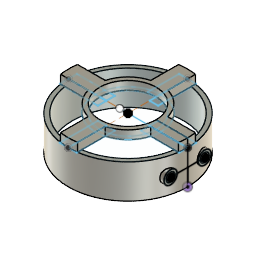
hexbug casing v6 (Autodesk Fusion 360 design; units mm, degrees)
Autodesk Fusion 360 part; units mm, degrees
sketch "Sketch1" plane through (0, 0, 0) normal (0, 0, 1) x (1, 0, 0)
  circle A0 centre (0, 0) radius 32.5
  circle A1 centre (0, 0) radius 35
  dimension "d1" = 65
  dimension "d2" = 70
  constraint coincident A0.centre A1.centre
  constraint concentric A0 A1
  measures "d1" diameter of A0
  measures "d2" diameter of A1
extrude "Extrude1" add sketch "Sketch1" along normal blind 20 makes body 1
sketch "Sketch2" plane through (0, 0, 0) normal (1, 0, 0) x (0, 1, 0)
  line L0 (0, 0) -> (0, 50)
  line L1 (0, 0) -> (0, 25)
  line L2 (0, 25) -> (-10, 25)
  circle A0 centre (-10, 25) radius 5
  line L3 (0, 25) -> (10, 25)
  circle A1 centre (10, 25) radius 5
  dimension "d5" = 50
  dimension "d7" = 10
  dimension "d8" = 10
  dimension "d9" = 10
  dimension "d10" = 10
  constraint coincident L0.start L1.start
  constraint vertical L0
  constraint midpoint L0 L1.end
  constraint perpendicular L0 L2
  constraint coincident L2.end A0.centre
  constraint perpendicular L1 L3
  constraint coincident L3.end A1.centre
  measures "d5" distance of L0.start L0.end
  measures "d7" distance of L1.end L2.end
  measures "d8" diameter of A0
  measures "d9" distance of L1.end L3.end
  measures "d10" diameter of A1
sketch "Sketch11" plane through (0, 0, 20) normal (0, 0, 1) x (-1, 0, 0)
  circle A0 centre (0, 0) radius 32.5
  circle A1 centre (0, 0) radius 35
  line L0 (0, -35) -> (5, -35)
  line L1 (4.424, 0) -> (0, 0)
  line L2 (-35, 0.0423) -> (0, 0)
  circle A2 centre (0, 0) radius 19.05 construction
  circle A3 centre (0, 0) radius 16.51 construction
  line L3 (0, 0) -> (0, 35) construction
  line L4 (35, 0) -> (0, 0) construction
  line L5 (0, 0) -> (0, -35) construction
  line L6 (35, 0) -> (12.7, 0) construction
  line L7 (12.7, 0) -> (12.7, 5) construction
  line L8 (12.7, 5) -> (35, 5) construction
  line L9 (35, 5) -> (35, 0) construction
  line L10 (35, 0) -> (12.7, 0) construction
  line L11 (12.7, 0) -> (12.7, -5) construction
  line L12 (12.7, -5) -> (35, -5) construction
  line L13 (35, -5) -> (35, 0) construction
  line L14 (0, 0) -> (5, 0) construction
  line L15 (5, -35) -> (0, -35) construction
  line L16 (0, -16.51) -> (5, -16.51)
  line L17 (5, -16.51) -> (5, -35)
  line L18 (5, -35) -> (0, -35)
  line L19 (0, -35) -> (0, -16.51)
  line L20 (0, -35) -> (-5, -35)
  line L21 (-5, -35) -> (-5, -12.7)
  line L22 (-5, -12.7) -> (0, -12.7)
  line L23 (0, -12.7) -> (0, -35)
  line L24 (0, 35) -> (5, 35)
  line L25 (5, 35) -> (5, 12.7)
  line L26 (5, 12.7) -> (0, 12.7)
  line L27 (0, 12.7) -> (0, 35)
  line L28 (0, 35) -> (-5, 35)
  line L29 (-5, 35) -> (-5, 12.7)
  line L30 (-5, 12.7) -> (0, 12.7)
  line L31 (0, 12.7) -> (0, 35)
  line L32 (-35, 0.0423) -> (-12.7, 0.0423)
  line L33 (-12.7, 0.0423) -> (-12.7, -4.9577)
  line L34 (-12.7, -4.9577) -> (-35, -4.9577)
  line L35 (-35, -4.9577) -> (-35, 0.0423)
  line L36 (-35, 0.0423) -> (-12.7, 0.0423)
  line L37 (-12.7, 0.0423) -> (-12.7, 5.0423)
  line L38 (-12.7, 5.0423) -> (-35, 5.0423)
  line L39 (-35, 5.0423) -> (-35, 0.0423)
  line L40 (35, 5) -> (12.7, 5)
  line L41 (12.7, 5) -> (12.7, 0)
  line L42 (12.7, 0) -> (35, 0)
  line L43 (35, 0) -> (35, 5)
  line L44 (35, 0) -> (12.7, 0)
  line L45 (12.7, 0) -> (12.7, -5)
  line L46 (12.7, -5) -> (35, -5)
  line L47 (35, -5) -> (35, 0)
  circle A4 centre (0, 0) radius 16.51
  circle A5 centre (0, 0) radius 19.05
  dimension "d39" = 38.1
  dimension "d40" = 33.02
  dimension "d41" = 5
  dimension "d42" = 5
  dimension "d43" = 5
  dimension "d44" = 5
  dimension "d45" = 22.3
  dimension "d46" = 22.3
  dimension "d47" = 22.3
  dimension "d48" = 5
  dimension "d49" = 22.3
  dimension "d50" = 5
  dimension "d51" = 5
  dimension "d52" = 22.3
  dimension "d53" = 5
  dimension "d54" = 22.3
  constraint horizontal L0
  constraint horizontal L1
  constraint coincident A1 L0.start
  constraint coincident A1 L2.start
  constraint coincident A0.centre A1.centre
  constraint concentric A2 A3
  constraint coincident A1 L3.end
  constraint perpendicular L1 L3
  constraint coincident A1 L4.start
  constraint perpendicular L3 L4
  constraint perpendicular L0 L5
  constraint horizontal L6
  constraint vertical L7
  constraint horizontal L8
  constraint vertical L9
  constraint horizontal L10
  constraint vertical L11
  constraint horizontal L12
  constraint vertical L13
  constraint horizontal L14
  constraint horizontal L15
  constraint horizontal L16
  constraint vertical L17
  constraint horizontal L18
  constraint vertical L19
  constraint coincident L5 L16.start
  constraint coincident A3 L16.start
  constraint horizontal L20
  constraint vertical L21
  constraint horizontal L22
  constraint vertical L23
  constraint horizontal L24
  constraint vertical L25
  constraint horizontal L26
  constraint vertical L27
  constraint horizontal L28
  constraint vertical L29
  constraint horizontal L30
  constraint vertical L31
  constraint horizontal L32
  constraint vertical L33
  constraint horizontal L34
  constraint vertical L35
  constraint horizontal L36
  constraint vertical L37
  constraint horizontal L38
  constraint vertical L39
  constraint horizontal L40
  constraint vertical L41
  constraint horizontal L42
  constraint vertical L43
  constraint horizontal L44
  constraint vertical L45
  constraint horizontal L46
  constraint vertical L47
  constraint coincident L16.start A4
  measures "d39" diameter of A2
  measures "d40" diameter of A3
  measures "d41" distance of L4.start L8.end
  measures "d42" distance of L4.start L12.end
  measures "d43" distance of L0.start L0.end
  measures "d44" distance of L0.start L20.end
  measures "d45" distance of L7.end L8.end
  measures "d46" distance of L20.end L21.end
  measures "d47" distance of L3.end L26.end
  measures "d48" distance of L3.end L24.end
  measures "d49" distance of L3.end L26.end
  measures "d50" distance of L3.end L28.end
  measures "d51" distance of L2.start L34.end
  measures "d52" distance of L33.end L34.end
  measures "d53" distance of L2.start L38.end
  measures "d54" distance of L37.end L38.end
extrude "Extrude17" add sketch "Sketch11" along normal blind 5 separate body contours A0 L40 L42 L44 A5 | A0 A1 L42 L44 L46 | A0 L42 L44 L46 A5 | A0 A1 L40 L42 L44 | L42 L44 L46 A4 A5 | L40 L42 L44 A4 A5 | A0 L25 L27 L31 A5 | A0 A1 L25 L27 L31 | L25 L40 A4 A5 | A0 A1 L17 L19 L23 | A0 L17 L19 L23 A5 | L16 L17 L46 A4 A5 | A0 L27 L29 L31 A5 | A0 A1 L27 L29 L31 | L25 L27 L31 A4 A5 | A0 A1 L19 L21 L23 | A0 L19 L21 L23 A5 | L16 L17 L19 L23 A5 | L27 L29 L31 A4 A5 | L19 L21 L23 A4 A5 | A0 L32 L36 L38 A5 | A0 A1 L2 L32 L36 L38 | L29 L38 A4 A5 | A0 A1 L2 L32 L34 L36 | A0 L2 L34 A5 | L21 L34 A4 A5 | L32 L36 L38 A4 A5 | L2 L34 A4 A5 makes body 2
ref_plane "WorkPlane3" through (35, 0, 0) normal (1, 0, 0) x (0, 1, 0)
sketch "Sketch12" plane through (35, 0, 0) normal (1, 0, 0) x (0, 1, 0)
  line L0 (0, 0) -> (0, 20)
  line L1 (0, 0) -> (0, 10)
  line L2 (0, 10) -> (10, 10)
  line L3 (0, 10) -> (-10, 10)
  circle A0 centre (-10, 10) radius 2.54
  circle A1 centre (-10, 10) radius 3.81
  circle A2 centre (10, 10) radius 2.54
  circle A3 centre (10, 10) radius 3.81
  dimension "d74" = 20
  dimension "d75" = 10
  dimension "d76" = 10
  dimension "d77" = 5.08
  dimension "d78" = 7.62
  dimension "d79" = 5.08
  dimension "d80" = 7.62
  constraint coincident L0.start L1.start
  constraint vertical L0
  constraint midpoint L0 L1.end
  constraint perpendicular L1 L2
  constraint perpendicular L1 L3
  constraint coincident L3.end A0.centre
  constraint concentric A0 A1
  constraint coincident L2.end A2.centre
  constraint concentric A2 A3
  measures "d74" distance of L0.start L0.end
  measures "d75" distance of L1.end L2.end
  measures "d76" distance of L1.end L3.end
  measures "d77" diameter of A0
  measures "d78" diameter of A1
  measures "d79" diameter of A2
  measures "d80" diameter of A3
extrude "Extrude18" add sketch "Sketch12" against normal blind 2.5 contours A1 bodies 1
extrude "Extrude19" add sketch "Sketch12" against normal blind 2.5 contours A3 bodies 1
ref_plane "WorkPlane4" through (-35, 0, 0) normal (1, 0, 0) x (0, 1, 0)
sketch "Sketch13" plane through (-35, 0, 0) normal (1, 0, 0) x (0, 1, 0)
  line L0 (0, 0) -> (0, 20)
  line L1 (0, 0) -> (0, 10)
  line L2 (0, 10) -> (-10, 10)
  line L3 (0, 10) -> (10, 10)
  circle A0 centre (10, 10) radius 2.54
  circle A1 centre (10, 10) radius 3.81
  circle A2 centre (-10, 10) radius 2.54
  circle A3 centre (-10, 10) radius 3.81
  dimension "d86" = 20
  dimension "d87" = 10
  dimension "d88" = 10
  dimension "d89" = 5.08
  dimension "d90" = 7.62
  dimension "d91" = 5.08
  dimension "d92" = 7.62
  constraint coincident L0.start L1.start
  constraint vertical L0
  constraint midpoint L0 L1.end
  constraint perpendicular L1 L2
  constraint perpendicular L1 L3
  constraint coincident L3.end A0.centre
  constraint concentric A0 A1
  constraint coincident L2.end A2.centre
  constraint concentric A2 A3
  measures "d86" distance of L0.start L0.end
  measures "d87" distance of L1.end L2.end
  measures "d88" distance of L1.end L3.end
  measures "d89" diameter of A0
  measures "d90" diameter of A1
  measures "d91" diameter of A2
  measures "d92" diameter of A3
extrude "Extrude20" add sketch "Sketch13" along normal blind 2.5 bodies 1
extrude "Extrude9" [suppressed]
extrude "Extrude10" [suppressed]
extrude "Extrude11" [suppressed]
extrude "Extrude12" [suppressed]
extrude "Extrude13" [suppressed]
extrude "Extrude14" [suppressed]
extrude "Extrude15" [suppressed]
extrude "Extrude16" [suppressed]
extrude "Extrude2" [suppressed]
sketch "Sketch3" plane through (0, 0, 0) normal (0, 1, 0) x (1, 0, 0)
  line L0 (0, 0) -> (0, -25)
  circle A0 centre (0, -25) radius 3.75
  dimension "d13" = 25
  dimension "d14" = 7.5
  constraint coincident L0.start origin
  constraint vertical L0
  constraint coincident L0.end A0.centre
  measures "d13" distance of L0.start L0.end
  measures "d14" diameter of A0
extrude "Extrude3" [suppressed]
sketch "Sketch4" plane through (35, 0, 0) normal (1, 0, 0) x (0, 1, 0)
  circle A0 centre (-10, 25) radius 5
  circle A1 centre (-10, 25) radius 3.75
  dimension "d17" = 7.5
  constraint concentric A0 A1
  measures "d17" diameter of A1
extrude "Extrude4" [suppressed]
extrude "Extrude5" [suppressed]
sketch "Sketch6" plane through (0, 0, 0) normal (1, 0, 0) x (0, 1, 0)
ref_plane "WorkPlane1" through (35, 0, 0) normal (1, 0, 0) x (0, 1, 0)
sketch "Sketch7" plane through (35, 0, 0) normal (1, 0, 0) x (0, 1, 0)
  line L0 (0, 0) -> (0, 20)
  circle A0 centre (0, 10) radius 5
  dimension "d25" = 20
  dimension "d26" = 10
  constraint coincident L0.start origin
  constraint vertical L0
  constraint midpoint L0 A0.centre
  measures "d25" distance of L0.start L0.end
  measures "d26" diameter of A0
extrude "Extrude6" [suppressed]
extrude "Extrude7" [suppressed]
ref_plane "WorkPlane2" through (60, 0, 0) normal (1, 0, 0) x (0, 1, 0)
sketch "Sketch8" plane through (60, 0, 0) normal (1, 0, 0) x (0, 1, 0)
sketch "Sketch9" plane through (0, 0, 0) normal (0, 0, 1) x (1, 0, 0)
sketch "Sketch10" plane through (0, 0, 0) normal (0, 0, 1) x (1, 0, 0)
  line L0 (0, 0) -> (-75, 0)
  circle A0 centre (-75, 0) radius 30
  circle A1 centre (-75, 0) radius 35
  dimension "d34" = 75
  dimension "d35" = 60
  dimension "d36" = 70
  constraint coincident L0.start origin
  constraint horizontal L0
  constraint coincident L0.end A0.centre
  constraint concentric A0 A1
  measures "d34" distance of L0.start L0.end
  measures "d35" diameter of A0
  measures "d36" diameter of A1
delete_face "DeleteFace1" [suppressed]
